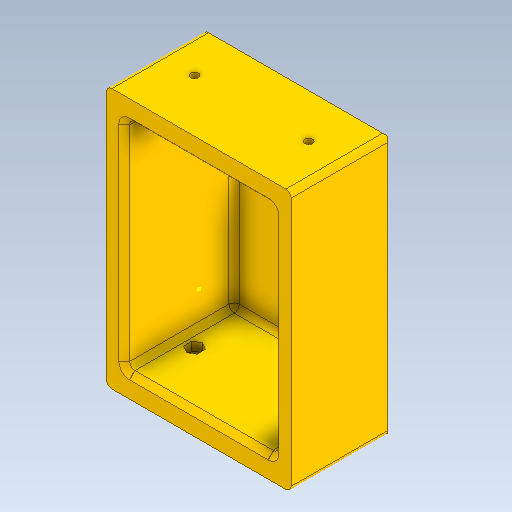
# Autodesk Inventor part: SuperBAndrenaHolder
Saved by Autodesk Inventor 2021 (Build 250183000, 183)
## iProperties
Created: 2020-10-25
Part Number: SuperBAndrenaHolder
Material: Generic
Document SubType Name: Modeling
Designer: lgnds
Density: 1 g/cm^3
Appearance: Default
Author: lgnds
Autodesk Inventor part; units mm, degrees
ref_plane "YZ Plane" through (0, 0, 0) normal (1, 0, 0) x (0, 1, 0)
ref_plane "XZ Plane" through (0, 0, 0) normal (0, 1, 0) x (-1, 0, 0)
ref_plane "XY Plane" through (0, 0, 0) normal (0, 0, 1) x (1, 0, 0)
sketch "Sketch1" plane through (0, 0, 0) normal (0, 0, 1) x (1, 0, 0)
  line L0 (-42.5, -61.5) -> (42.5, -61.5)
  line L1 (42.5, -61.5) -> (42.5, 61.5)
  line L2 (42.5, 61.5) -> (-42.5, 61.5)
  line L3 (-42.5, 61.5) -> (-42.5, -61.5)
  line L4 (-42.5, -61.5) -> (42.5, 61.5) construction
  line L5 (42.5, -61.5) -> (-42.5, 61.5) construction
  line L6 (-52.5, -74) -> (52.5, -74)
  line L7 (52.5, -74) -> (52.5, 74)
  line L8 (52.5, 74) -> (-52.5, 74)
  line L9 (-52.5, 74) -> (-52.5, -74)
  line L10 (-52.5, -74) -> (52.5, 74) construction
  line L11 (52.5, -74) -> (-52.5, 74) construction
  point P0 (0, 0)
  dimension "d0" = 85
  dimension "d1" = 123
  dimension "d2" = 10
  dimension "d4" = 148
  constraints: 24 end point, 4 midpoint, 4 parallel, 2 horizontal, 2 perpendicular
  measures "d0" distance of L1.end L2.end
  measures "d1" distance of L0.end L1.end
  measures "d2" distance between parallel lines of L3 L9
  measures "d4" distance between parallel lines of L6 L8
extrude "Extrusion1" add sketch "Sketch1" along normal blind 60
sketch "Sketch2" plane through (0, 0, 0) normal (0, 0, -1) x (-1, 0, 0)
  line L0 (-52.5, -74) -> (-52.5, 74) projected
  line L1 (52.5, -74) -> (-52.5, -74) projected
  line L2 (52.5, 74) -> (52.5, -74) projected
  line L3 (-52.5, 74) -> (52.5, 74) projected
  line L4 (42.5, -61.5) -> (42.5, 61.5) projected
  line L5 (-42.5, -61.5) -> (42.5, -61.5) projected
  line L6 (-42.5, 61.5) -> (-42.5, -61.5) projected
  line L7 (42.5, 61.5) -> (-42.5, 61.5) projected
  point P0 (0, 0)
extrude "Extrusion2" add sketch "Sketch2" along normal blind 5 contours L0 L3 L2 L1 | L5 L6 L7 L4
chamfer "Chamfer1" distance 10 angle 45 4 edges at (0, -74, -5) (0, 74, -5) (52.5, 0, -5) (-52.5, 0, -5)
draft "FaceDraft1" angle 2.5 pull direction (0, 0, 1) faces at (-14.1667, 61.5, 20) fixed edges at (0, 61.5, 60)
draft "FaceDraft2" angle 2.5 pull direction (0, 0, 1) faces at (-42.5, 19.6268, 40) fixed edges at (-42.5, 0, 60)
draft "FaceDraft3" angle 2.5 pull direction (0, 0, 1) faces at (-13.2934, -61.5, 40) fixed edges at (0, -61.5, 60)
draft "FaceDraft4" angle 2.5 pull direction (0, 0, 1) faces at (42.5, -19.6268, 40) fixed edges at (42.5, 0, 60)
fillet "Fillet1" radius 3 8 edges at (-41.1902, 60.1902, 30) (41.1902, 60.1902, 30) (41.1902, -60.1902, 30) (-41.1902, -60.1902, 30) (-39.8803, 0, 0) (0, -58.8803, 0) (39.8803, 0, 0) (0, 58.8803, 0)
fillet "Fillet2" radius 3 4 edges at (52.5, -74, 32.5) (-52.5, -74, 32.5) (52.5, 74, 32.5) (-52.5, 74, 32.5)
sketch "Sketch3" plane through (-49.5, -74, 5) normal (0, -1, 0) x (1, 0, 0)
  circle A0 centre (17, 25) radius 2.25
  line L0 (-3, 55) -> (-3, 0) projected
  line L1 (0, 55) -> (99, 55) construction
  line L2 (49.5, 68) -> (49.5, -23) projected
  circle A1 centre (82, 25) radius 2.25
  point P0 (49.5, -5)
  dimension "d18" = 20
  dimension "d19" = 30
  dimension "d20" = 4.5
  constraints: 2 centre point, 1 symmetric about line, 1 other
  measures "d18" distance from line of L0 A0.centre
  measures "d19" distance from line of L1 A0.centre
  measures "d20" diameter of A0
extrude "Extrusion3" cut sketch "Sketch3" against normal up to surface (148 mm away)
sketch "Sketch4" plane through (-39.5029, -61.5, 60) normal (0, 0.9990482, 0.0436194) x (1, 0, 0)
  ellipse E0 centre (72.0029, 30.0286) end of major axis (72.0029, 32.2807) minor radius 2.25 projected
  ellipse E1 centre (7.0029, 30.0286) end of major axis (7.0029, 32.2807) minor radius 2.25 projected
  line L0 (39.5029, 85.1273) -> (39.5029, -14.824) projected
  line L1 (10.9029, 32.2802) -> (10.9029, 27.7769)
  line L2 (10.9029, 27.7769) -> (7.0029, 25.5252)
  line L3 (7.0029, 25.5252) -> (3.1029, 27.7769)
  line L4 (3.1029, 27.7769) -> (3.1029, 32.2802)
  line L5 (3.1029, 32.2802) -> (7.0029, 34.5319)
  line L6 (7.0029, 34.5319) -> (10.9029, 32.2802)
  point P0 (39.5029, 62.6255)
  dimension "d23" = 7.8
  constraints: 12 end point, 1 coincident, 1 vertical, 15 other
  measures "d23" distance between parallel lines of L6 L3
extrude "Extrusion4" cut sketch "Sketch4" against normal blind 5 contours E1 | L1 L2 L3 L4 L5 L6
mirror "Mirror1" about plane through (0, 0, 0) normal (1, 0, 0) of "Extrusion4"
mirror "Mirror2" about plane through (0, 0, 0) normal (0, 1, 0) of "Extrusion4", "Mirror1"
sketch "Sketch5" plane through (0, 0, 60) normal (0, 0, 1) x (1, 0, 0)
  point P0 (0, 0)
chamfer "Chamfer2" distance 3 angle 45 8 edges at (42.5, 0, 60) (41.6225, -60.6225, 60) (0, -61.5, 60) (-41.6225, -60.6225, 60) (-42.5, 0, 60) (-41.6225, 60.6225, 60) (0, 61.5, 60) (41.6225, 60.6225, 60)
body "Solid1"
